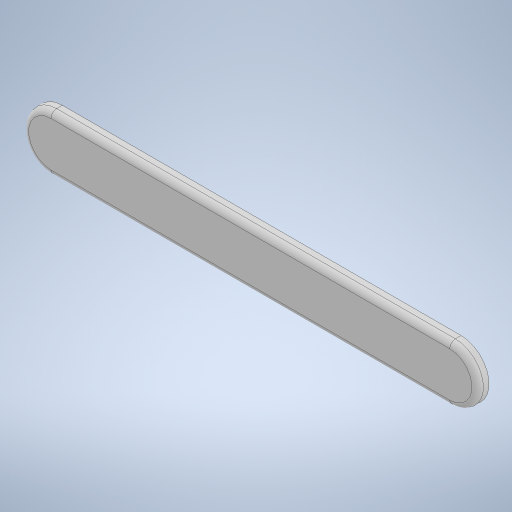
# Autodesk Inventor part: foot
Saved by Autodesk Inventor 2024 (Build 280153000, 153)
## iProperties
Created: 2023-08-03
Part Number: foot
Material: Generic
Document SubType Name: Modeling
Designer: Mika
Density: 1 g/cm^3
Appearance: Default
Author: Mika
Autodesk Inventor part; units mm, degrees
ref_plane "YZ Plane" through (0, 0, 0) normal (1, 0, 0) x (0, 1, 0)
ref_plane "XZ Plane" through (0, 0, 0) normal (0, 1, 0) x (-1, 0, 0)
ref_plane "XY Plane" through (0, 0, 0) normal (0, 0, 1) x (1, 0, 0)
sketch "Sketch1" plane through (0, 0, 0) normal (0, 0, 1) x (1, 0, 0)
  line L0 (0, 0) -> (69.8, 0) construction
  line L1 (0, -4.9) -> (69.8, -4.9)
  line L2 (69.8, 4.9) -> (0, 4.9)
  arc A0 (0, 4.9) -> (0, -4.9) centre (0, 0) ccw
  arc A1 (69.8, -4.9) -> (69.8, 4.9) centre (69.8, 0) ccw
  point P0 (34.9, 0)
  dimension "d0" = 69.8
  dimension "d1" = 9.8
  constraints: 8 end point, 4 point on circle, 4 tangent, 2 centre point, 1 horizontal, 1 midpoint, 1 parallel
  measures "d0" distance of L0.start L0.end
  measures "d1" diameter of A1
extrude "Extrusion1" add sketch "Sketch1" along normal blind 2
fillet "Fillet1" radius 1 4 edges at (-4.9, 0, 2) (34.9, -4.9, 2) (74.7, 0, 2) (34.9, 4.9, 2)
body "Solid1"
